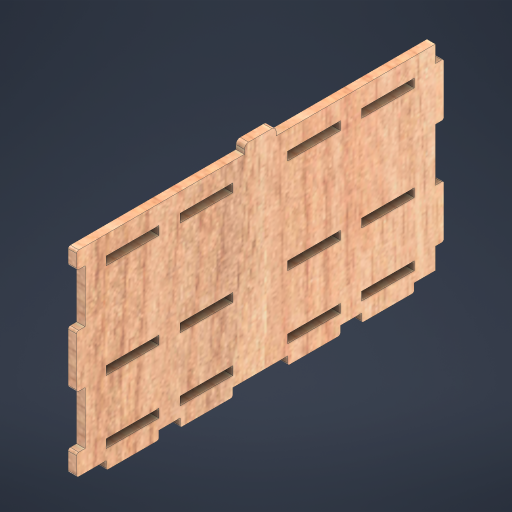
# Autodesk Inventor part: Side
Saved by Autodesk Inventor 2024.1 (Build 281209000, 209)
## iProperties
Created: 2024-05-23
Part Number: Side
Material: Wood (Birch)
Document SubType Name: Modeling
Designer: Tim Jäger
Density: 0.55 g/cm^3
Appearance: Birch - Natural Polished
Author: Tim Jäger
Autodesk Inventor part; units mm, degrees
ref_plane "YZ Plane" through (0, 0, 0) normal (1, 0, 0) x (0, 1, 0)
ref_plane "XZ Plane" through (0, 0, 0) normal (0, 1, 0) x (-1, 0, 0)
ref_plane "XY Plane" through (0, 0, 0) normal (0, 0, 1) x (1, 0, 0)
sketch "Sketch1" plane through (0, 0, 0) normal (1, 0, 0) x (0, 1, 0)
  line L0 (79, 73) -> (75, 73)
  line L1 (75, 73) -> (75, 48)
  line L2 (75, 48) -> (79, 48)
  line L3 (79, 48) -> (79, 73)
  line L4 (79, 38) -> (75, 38)
  line L5 (75, 38) -> (75, 13)
  line L6 (75, 13) -> (79, 13)
  line L7 (79, 13) -> (79, 38)
  line L8 (-29.2828, 0) -> (112.6971, 0) construction
  line L9 (79, -73) -> (75, -73)
  line L10 (75, -73) -> (75, -48)
  line L11 (75, -48) -> (79, -48)
  line L12 (79, -48) -> (79, -73)
  line L13 (79, -38) -> (75, -38)
  line L14 (75, -38) -> (75, -13)
  line L15 (75, -13) -> (79, -13)
  line L16 (79, -13) -> (79, -38)
  line L17 (0, 13) -> (4, 13)
  line L18 (4, 38) -> (0, 38)
  line L19 (0, 38) -> (0, 13)
  line L20 (0, 48) -> (4, 48)
  line L21 (4, 73) -> (0, 73)
  line L22 (0, 73) -> (0, 48)
  line L23 (4, 48) -> (4, 73)
  line L24 (4, 13) -> (4, 38)
  line L25 (0, -13) -> (4, -13)
  line L26 (4, -13) -> (4, -38)
  line L27 (0, -38) -> (0, -13)
  line L28 (0, -48) -> (4, -48)
  line L29 (4, -73) -> (0, -73)
  line L30 (4, -48) -> (4, -73)
  line L31 (0, -73) -> (0, -48)
  line L32 (4, -38) -> (0, -38)
  line L33 (30, 13) -> (34, 13)
  line L34 (30, 38) -> (30, 13)
  line L35 (34, 13) -> (34, 38)
  line L36 (34, 38) -> (30, 38)
  line L37 (34, -73) -> (30, -73)
  line L38 (30, -73) -> (30, -48)
  line L39 (30, -48) -> (34, -48)
  line L40 (34, -48) -> (34, -73)
  line L41 (30, -38) -> (30, -13)
  line L42 (34, -38) -> (30, -38)
  line L43 (34, -13) -> (34, -38)
  line L44 (30, -13) -> (34, -13)
  line L45 (34, 73) -> (30, 73)
  line L46 (30, 73) -> (30, 48)
  line L47 (30, 48) -> (34, 48)
  line L48 (34, 48) -> (34, 73)
  line L49 (88, 83) -> (-5, 83)
  line L50 (-5, 83) -> (-5, -83)
  line L51 (-5, -83) -> (88, -83)
  line L52 (88, -83) -> (88, 83)
  line L53 (80, -83) -> (55, -83)
  line L54 (55, -83) -> (55, -87)
  line L55 (55, -87) -> (80, -87)
  line L56 (80, -87) -> (80, -83)
  line L57 (5, -87) -> (30, -87)
  line L58 (30, -87) -> (30, -83)
  line L59 (30, -83) -> (5, -83)
  line L60 (5, -83) -> (5, -87)
  line L61 (-5, -13) -> (-5, -38)
  line L62 (-9, -13) -> (-5, -13)
  line L63 (-9, -38) -> (-9, -13)
  line L64 (-9, 48) -> (-5, 48)
  line L65 (-9, 73) -> (-9, 48)
  line L66 (-5, 73) -> (-9, 73)
  line L67 (-5, 48) -> (-5, 73)
  line L68 (-5, -38) -> (-9, -38)
  line L69 (-5, -73) -> (-9, -73)
  line L70 (-5, -48) -> (-5, -73)
  line L71 (-9, -73) -> (-9, -48)
  line L72 (-9, -48) -> (-5, -48)
  line L73 (-9, 13) -> (-5, 13)
  line L74 (-5, 13) -> (-5, 38)
  line L75 (-5, 38) -> (-9, 38)
  line L76 (-9, 38) -> (-9, 13)
  line L77 (88, 7.5) -> (90, 7.5)
  line L78 (92, 5.5) -> (92, -5.5)
  line L79 (90, -7.5) -> (88, -7.5)
  line L80 (88, -7.5) -> (88, 7.5)
  arc A0 (92, 5.5) -> (90, 7.5) centre (90, 5.5) ccw
  arc A1 (90, -7.5) -> (92, -5.5) centre (90, -5.5) ccw
  line L81 (88, 87) -> (80, 87)
  line L82 (80, 87) -> (80, 83)
  line L83 (80, 83) -> (88, 83)
  line L84 (88, 83) -> (88, 87)
  line L85 (-5, 83) -> (5, 83)
  line L86 (5, 83) -> (5, 87)
  line L87 (5, 87) -> (-5, 87)
  line L88 (-5, 87) -> (-5, 83)
  line L89 (30, 83) -> (55, 83)
  line L90 (55, 83) -> (55, 87)
  line L91 (55, 87) -> (30, 87)
  line L92 (30, 87) -> (30, 83)
  point P0 (0, 0)
  point P1 (77, 73)
  point P2 (77, -73)
  point P3 (2, 73)
  point P4 (2, -73)
  point P5 (32, -73)
  point P6 (32, 73)
  point P7 (5, -85)
  point P8 (-9, 0)
  point P9 (-7, 73)
  point P10 (-7, -73)
  point P11 (-5, 38)
  point P12 (-5, -38)
  point P13 (92, -7.5)
  point P14 (92, 7.5)
  point P15 (92, 0)
  point P16 (-5, 38)
  point P17 (-5, -38)
  point P18 (-5, 83)
  dimension "d0" = 4
  dimension "d1" = 25
  dimension "d2" = 25
  dimension "d3" = 10
  dimension "d4" = 4
  dimension "d5" = 13
  dimension "d14" = 75
  dimension "d17" = 75
  dimension "d24" = 45
  dimension "d29" = 9
  dimension "d30" = 5
  dimension "d31" = 10
  dimension "d32" = 10
  dimension "d33" = 25
  dimension "d34" = 25
  dimension "d35" = 25
  dimension "d36" = 10
  dimension "d39" = 9
  dimension "d46" = 15
  dimension "d47" = 4
  dimension "d48" = 2
  dimension "d49" = 2
  constraints: 184 end point, 18 parallel, 12 horizontal, 10 point on line, 9 perpendicular, 9 symmetric about line, 6 vertical alignment, 5 equal length, 4 point on circle, 4 tangent, 3 collinear, 3 midpoint, 2 centre point, 100 other
  measures "d0" distance of L2.end L1.end
  measures "d1" distance of L1.end L0.end
  measures "d2" distance of L5.end L4.end
  measures "d3" distance of L2.end L4.start
  measures "d4" distance of L5.end L6.end
  measures "d5" vertical distance of L5.end point (0, 0)
  measures "d14" distance from line of point (0, 0) L1
  measures "d17" distance of L0.start L21.start
  measures "d24" distance of L4.start L35.end
  measures "d29" distance between parallel lines of L3 L52
  measures "d30" distance between parallel lines of L19 L50
  measures "d31" distance between parallel lines of L9 L51
  measures "d32" distance between parallel lines of L49 L0
  measures "d33" distance between parallel lines of L58 L54
  measures "d34" distance of L54.end L55.end
  measures "d35" distance of L57.start L57.end
  measures "d36" distance from line of L50 point (5, -85)
  measures "d39" distance of L25.end L61.start
  measures "d46" distance of point (92, 7.5) point (92, -7.5)
  measures "d47" distance of point (92, -7.5) L79.end
  measures "d48" radius of A0
  measures "d49" radius of A1
extrude "Extrusion1" add sketch "Sketch1" along normal blind 4
fillet "Fillet1" radius 1 18 edges at (2, 88, 87) (2, 80, 87) (2, 55, 87) (2, 30, 87) (2, 5, 87) (2, -5, 87) (2, -9, 73) (2, -9, 38) (2, -9, -13) (2, -9, 48) (2, -9, 13) (2, -9, -38) (2, -9, -48) (2, -9, -73) (2, 5, -87) (2, 30, -87) (2, 55, -87) (2, 80, -87)
body "Solid1"
